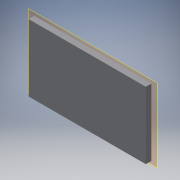
# Autodesk Inventor part: tpu pad 2
Saved by Autodesk Inventor 2019.4 (Build 234330000, 330)
## iProperties
Created: 2021-04-16
Part Number: tpu pad 2
Material: Generic
Document SubType Name: Modeling
Designer: Ian
Density: 1 g/cm^3
Appearance: Default
Author: Ian
Autodesk Inventor part; units mm, degrees
ref_plane "YZ Plane" through (0, 0, 0) normal (1, 0, 0) x (0, 1, 0)
ref_plane "XZ Plane" through (0, 0, 0) normal (0, 1, 0) x (-1, 0, 0)
ref_plane "XY Plane" through (0, 0, 0) normal (0, 0, 1) x (1, 0, 0)
ref_plane "Work Plane1" through (0, 0, 0) normal (0, 0, 1) x (1, 0, 0)
sketch "Sketch1" plane through (0, 0, 0) normal (0, 0, 1) x (1, 0, 0)
  line L0 (-42, 0) -> (0, 0) projected
  line L1 (-42, 0) -> (-42, -24) projected
  line L2 (0, -24) -> (-42, -24) projected
  line L3 (0, 0) -> (0, -24) projected
extrude "Extrusion1" add sketch "Sketch1" along normal blind 2
body "Solid1"
